Autodesk Fusion 360 part; units mm, degrees
(part 5 of 6)
sketch "Gear Tooth (2)" plane through (0, 0, 0) normal (0, 0, 1) x (1, 0, 0)
  spline S0 degree 5 poles (33.47, -4.9149) (33.4943, -4.9185) (33.543, -4.9249) (33.6161, -4.932) (33.714, -4.9371) (33.8368, -4.9373) (33.96, -4.9332) (34.0834, -4.9264) (34.2068, -4.9182) (34.3304, -4.9091) (34.454, -4.8988) (34.5776, -4.8871) (34.7013, -4.8735) (34.8251, -4.8577) (34.949, -4.8398) (35.0728, -4.8198) (35.1967, -4.7983) (35.3206, -4.7752) (35.4445, -4.751) (35.5683, -4.7256) (35.6921, -4.699) (35.8159, -4.6711) (35.9396, -4.6419) (36.0632, -4.6113) (36.1868, -4.5793) (36.3104, -4.5461) (36.4339, -4.5117) (36.5573, -4.4761) (36.6806, -4.4394) (36.8038, -4.4016) (36.927, -4.3627) (37.05, -4.3226) (37.173, -4.2815) (37.2958, -4.2393) (37.4185, -4.1961) (37.5411, -4.1517) (37.6636, -4.1064) (37.7859, -4.06) (37.9082, -4.0126) (38.0302, -3.9642) (38.1522, -3.9148) (38.274, -3.8645) (38.3956, -3.8132) (38.5172, -3.7609) (38.6385, -3.7077) (38.7597, -3.6535) (38.8807, -3.5984) (39.0016, -3.5424) (39.1223, -3.4854) (39.2428, -3.4276) (39.3631, -3.3689) (39.4833, -3.3092) (39.6032, -3.2487) (39.723, -3.1873) (39.8426, -3.125) (39.962, -3.0619) (40.0812, -2.9979) (40.2002, -2.9331) (40.319, -2.8674) (40.4376, -2.8009) (40.5559, -2.7335) (40.6741, -2.6653) (40.792, -2.5963) (40.9098, -2.5265) (41.0273, -2.4559) (41.1445, -2.3844) (41.2616, -2.3122) (41.3783, -2.2392) (41.4949, -2.1654) (41.6112, -2.0908) (41.7273, -2.0154) (41.82, -1.9545) (41.8894, -1.9084) (41.9356, -1.8776) (41.9587, -1.8621) knots 0 0 0 0 0 0 0.01428571 0.02857143 0.04285714 0.05714286 0.07142857 0.08571429 0.1 0.11428571 0.12857143 0.14285714 0.15714286 0.17142857 0.18571429 0.2 0.21428571 0.22857143 0.24285714 0.25714286 0.27142857 0.28571429 0.3 0.31428571 0.32857143 0.34285714 0.35714286 0.37142857 0.38571429 0.4 0.41428571 0.42857143 0.44285714 0.45714286 0.47142857 0.48571429 0.5 0.51428571 0.52857143 0.54285714 0.55714286 0.57142857 0.58571429 0.6 0.61428571 0.62857143 0.64285714 0.65714286 0.67142857 0.68571429 0.7 0.71428571 0.72857143 0.74285714 0.75714286 0.77142857 0.78571429 0.8 0.81428571 0.82857143 0.84285714 0.85714286 0.87142857 0.88571429 0.9 0.91428571 0.92857143 0.94285714 0.95714286 0.97142857 0.98571429 1 1 1 1 1 1
  spline S1 degree 5 poles (33.47, 4.9149) (33.4943, 4.9185) (33.543, 4.9249) (33.6161, 4.932) (33.714, 4.9371) (33.8368, 4.9373) (33.96, 4.9332) (34.0834, 4.9264) (34.2068, 4.9182) (34.3304, 4.9091) (34.454, 4.8988) (34.5776, 4.8871) (34.7013, 4.8735) (34.8251, 4.8577) (34.949, 4.8398) (35.0728, 4.8198) (35.1967, 4.7983) (35.3206, 4.7752) (35.4445, 4.751) (35.5683, 4.7256) (35.6921, 4.699) (35.8159, 4.6711) (35.9396, 4.6419) (36.0632, 4.6113) (36.1868, 4.5793) (36.3104, 4.5461) (36.4339, 4.5117) (36.5573, 4.4761) (36.6806, 4.4394) (36.8038, 4.4016) (36.927, 4.3627) (37.05, 4.3226) (37.173, 4.2815) (37.2958, 4.2393) (37.4185, 4.1961) (37.5411, 4.1517) (37.6636, 4.1064) (37.7859, 4.06) (37.9082, 4.0126) (38.0302, 3.9642) (38.1522, 3.9148) (38.274, 3.8645) (38.3956, 3.8132) (38.5172, 3.7609) (38.6385, 3.7077) (38.7597, 3.6535) (38.8807, 3.5984) (39.0016, 3.5424) (39.1223, 3.4854) (39.2428, 3.4276) (39.3631, 3.3689) (39.4833, 3.3092) (39.6032, 3.2487) (39.723, 3.1873) (39.8426, 3.125) (39.962, 3.0619) (40.0812, 2.9979) (40.2002, 2.9331) (40.319, 2.8674) (40.4376, 2.8009) (40.5559, 2.7335) (40.6741, 2.6653) (40.792, 2.5963) (40.9098, 2.5265) (41.0273, 2.4559) (41.1445, 2.3844) (41.2616, 2.3122) (41.3783, 2.2392) (41.4949, 2.1654) (41.6112, 2.0908) (41.7273, 2.0154) (41.82, 1.9545) (41.8894, 1.9084) (41.9356, 1.8776) (41.9587, 1.8621) knots 0 0 0 0 0 0 0.01428571 0.02857143 0.04285714 0.05714286 0.07142857 0.08571429 0.1 0.11428571 0.12857143 0.14285714 0.15714286 0.17142857 0.18571429 0.2 0.21428571 0.22857143 0.24285714 0.25714286 0.27142857 0.28571429 0.3 0.31428571 0.32857143 0.34285714 0.35714286 0.37142857 0.38571429 0.4 0.41428571 0.42857143 0.44285714 0.45714286 0.47142857 0.48571429 0.5 0.51428571 0.52857143 0.54285714 0.55714286 0.57142857 0.58571429 0.6 0.61428571 0.62857143 0.64285714 0.65714286 0.67142857 0.68571429 0.7 0.71428571 0.72857143 0.74285714 0.75714286 0.77142857 0.78571429 0.8 0.81428571 0.82857143 0.84285714 0.85714286 0.87142857 0.88571429 0.9 0.91428571 0.92857143 0.94285714 0.95714286 0.97142857 0.98571429 1 1 1 1 1 1
  arc A0 (41.9587, -1.8621) -> (41.9587, 1.8621) centre (0, 0) ccw
  line L0 (28.7398, -4.2203) -> (33.47, -4.9149)
  line L1 (28.7398, 4.2203) -> (33.47, 4.9149)
  line L2 (28.7398, -4.2203) -> (28.7398, 4.2203)
  point P0 (34.058, -4.9275)
  point P1 (34.6545, -4.8784)
  point P2 (35.2564, -4.787)
  point P3 (35.862, -4.66)
  point P4 (36.4705, -4.5009)
  point P5 (37.0809, -4.3121)
  point P6 (37.6927, -4.0952)
  point P7 (38.305, -3.8513)
  point P8 (38.9173, -3.5813)
  point P9 (39.5291, -3.286)
  point P10 (40.1396, -2.966)
  point P11 (40.7485, -2.6217)
  point P12 (41.355, -2.2536)
  point P13 (34.058, 4.9275)
  point P14 (34.6545, 4.8784)
  point P15 (35.2564, 4.787)
  point P16 (35.862, 4.66)
  point P17 (36.4705, 4.5009)
  point P18 (37.0809, 4.3121)
  point P19 (37.6927, 4.0952)
  point P20 (38.305, 3.8513)
  point P21 (38.9173, 3.5813)
  point P22 (39.5291, 3.286)
  point P23 (40.1396, 2.966)
  point P24 (40.7485, 2.6217)
  point P25 (41.355, 2.2536)
extrude "Extrude11" add sketch "Gear Tooth (2)" along normal blind 4 bodies 6
fillet "Fillet3" radius 2 2 edges at (28.7497, -4.2218, 2) (28.7497, 4.2218, 2) on bodies 6
pattern_circular "C-Pattern3" count 12 over 360 about axis through (0, 0, 0) along (0, 0, 1) of "Extrude11", "Fillet3"
sketch "Diametrial Pitch Circle (2)" plane through (0, 0, 0) normal (0, 0, 1) x (1, 0, 0)
  circle A0 centre (0, 0) radius 36 construction
sketch "Sketch15" plane through (0, 0, 0) normal (0, 0, 1) x (1, 0, 0)
  arc A0 (27.643, -8.9572) -> (28.4181, -6.0644) centre (0, 0) ccw
  arc A1 (30.6647, -4.503) -> (28.4181, -6.0644) centre (30.3741, -6.4818) ccw
  line L0 (30.6647, -4.503) -> (33.47, -4.9149)
  spline S0 degree 5 poles (33.47, -4.9149) (33.4943, -4.9185) (33.543, -4.9249) (33.6161, -4.932) (33.714, -4.9371) (33.8368, -4.9373) (33.96, -4.9332) (34.0834, -4.9264) (34.2068, -4.9182) (34.3304, -4.9091) (34.454, -4.8988) (34.5776, -4.8871) (34.7013, -4.8735) (34.8251, -4.8577) (34.949, -4.8398) (35.0728, -4.8198) (35.1967, -4.7983) (35.3206, -4.7752) (35.4445, -4.751) (35.5683, -4.7256) (35.6921, -4.699) (35.8159, -4.6711) (35.9396, -4.6419) (36.0632, -4.6113) (36.1868, -4.5793) (36.3104, -4.5461) (36.4339, -4.5117) (36.5573, -4.4761) (36.6806, -4.4394) (36.8038, -4.4016) (36.927, -4.3627) (37.05, -4.3226) (37.173, -4.2815) (37.2958, -4.2393) (37.4185, -4.1961) (37.5411, -4.1517) (37.6636, -4.1064) (37.7859, -4.06) (37.9082, -4.0126) (38.0302, -3.9642) (38.1522, -3.9148) (38.274, -3.8645) (38.3956, -3.8132) (38.5172, -3.7609) (38.6385, -3.7077) (38.7597, -3.6535) (38.8807, -3.5984) (39.0016, -3.5424) (39.1223, -3.4854) (39.2428, -3.4276) (39.3631, -3.3689) (39.4833, -3.3092) (39.6032, -3.2487) (39.723, -3.1873) (39.8426, -3.125) (39.962, -3.0619) (40.0812, -2.9979) (40.2002, -2.9331) (40.319, -2.8674) (40.4376, -2.8009) (40.5559, -2.7335) (40.6741, -2.6653) (40.792, -2.5963) (40.9098, -2.5265) (41.0273, -2.4559) (41.1445, -2.3844) (41.2616, -2.3122) (41.3783, -2.2392) (41.4949, -2.1654) (41.6112, -2.0908) (41.7273, -2.0154) (41.82, -1.9545) (41.8894, -1.9084) (41.9356, -1.8776) (41.9587, -1.8621) knots 0 0 0 0 0 0 0.01428571 0.02857143 0.04285714 0.05714286 0.07142857 0.08571429 0.1 0.11428571 0.12857143 0.14285714 0.15714286 0.17142857 0.18571429 0.2 0.21428571 0.22857143 0.24285714 0.25714286 0.27142857 0.28571429 0.3 0.31428571 0.32857143 0.34285714 0.35714286 0.37142857 0.38571429 0.4 0.41428571 0.42857143 0.44285714 0.45714286 0.47142857 0.48571429 0.5 0.51428571 0.52857143 0.54285714 0.55714286 0.57142857 0.58571429 0.6 0.61428571 0.62857143 0.64285714 0.65714286 0.67142857 0.68571429 0.7 0.71428571 0.72857143 0.74285714 0.75714286 0.77142857 0.78571429 0.8 0.81428571 0.82857143 0.84285714 0.85714286 0.87142857 0.88571429 0.9 0.91428571 0.92857143 0.94285714 0.95714286 0.97142857 0.98571429 1 1 1 1 1 1
  arc A2 (41.9587, -1.8621) -> (41.9587, 1.8621) centre (0, 0) ccw
  spline S1 degree 5 poles (41.9587, 1.8621) (41.9356, 1.8776) (41.8894, 1.9084) (41.82, 1.9545) (41.7273, 2.0154) (41.6112, 2.0908) (41.4949, 2.1654) (41.3783, 2.2392) (41.2616, 2.3122) (41.1445, 2.3844) (41.0273, 2.4559) (40.9098, 2.5265) (40.792, 2.5963) (40.6741, 2.6653) (40.5559, 2.7335) (40.4376, 2.8009) (40.319, 2.8674) (40.2002, 2.9331) (40.0812, 2.9979) (39.962, 3.0619) (39.8426, 3.125) (39.723, 3.1873) (39.6032, 3.2487) (39.4833, 3.3092) (39.3631, 3.3689) (39.2428, 3.4276) (39.1223, 3.4854) (39.0016, 3.5424) (38.8807, 3.5984) (38.7597, 3.6535) (38.6385, 3.7077) (38.5172, 3.7609) (38.3956, 3.8132) (38.274, 3.8645) (38.1522, 3.9148) (38.0302, 3.9642) (37.9082, 4.0126) (37.7859, 4.06) (37.6636, 4.1064) (37.5411, 4.1517) (37.4185, 4.1961) (37.2958, 4.2393) (37.173, 4.2815) (37.05, 4.3226) (36.927, 4.3627) (36.8038, 4.4016) (36.6806, 4.4394) (36.5573, 4.4761) (36.4339, 4.5117) (36.3104, 4.5461) (36.1868, 4.5793) (36.0632, 4.6113) (35.9396, 4.6419) (35.8159, 4.6711) (35.6921, 4.699) (35.5683, 4.7256) (35.4445, 4.751) (35.3206, 4.7752) (35.1967, 4.7983) (35.0728, 4.8198) (34.949, 4.8398) (34.8251, 4.8577) (34.7013, 4.8735) (34.5776, 4.8871) (34.454, 4.8988) (34.3304, 4.9091) (34.2068, 4.9182) (34.0834, 4.9264) (33.96, 4.9332) (33.8368, 4.9373) (33.714, 4.9371) (33.6161, 4.932) (33.543, 4.9249) (33.4943, 4.9185) (33.47, 4.9149) knots -1 -1 -1 -1 -1 -1 -0.98571429 -0.97142857 -0.95714286 -0.94285714 -0.92857143 -0.91428571 -0.9 -0.88571429 -0.87142857 -0.85714286 -0.84285714 -0.82857143 -0.81428571 -0.8 -0.78571429 -0.77142857 -0.75714286 -0.74285714 -0.72857143 -0.71428571 -0.7 -0.68571429 -0.67142857 -0.65714286 -0.64285714 -0.62857143 -0.61428571 -0.6 -0.58571429 -0.57142857 -0.55714286 -0.54285714 -0.52857143 -0.51428571 -0.5 -0.48571429 -0.47142857 -0.45714286 -0.44285714 -0.42857143 -0.41428571 -0.4 -0.38571429 -0.37142857 -0.35714286 -0.34285714 -0.32857143 -0.31428571 -0.3 -0.28571429 -0.27142857 -0.25714286 -0.24285714 -0.22857143 -0.21428571 -0.2 -0.18571429 -0.17142857 -0.15714286 -0.14285714 -0.12857143 -0.11428571 -0.1 -0.08571429 -0.07142857 -0.05714286 -0.04285714 -0.02857143 -0.01428571 0 0 0 0 0 0
  line L1 (33.47, 4.9149) -> (30.6647, 4.503)
  arc A3 (28.4181, 6.0644) -> (30.6647, 4.503) centre (30.3741, 6.4818) ccw
  arc A4 (28.4181, 6.0644) -> (27.643, 8.9572) centre (0, 0) ccw
  arc A5 (28.8079, 11.4326) -> (27.643, 8.9572) centre (29.5456, 9.5737) ccw
  line L2 (28.8079, 11.4326) -> (31.4433, 12.4785)
  spline S2 degree 5 poles (31.4433, 12.4785) (31.4662, 12.4876) (31.5115, 12.5064) (31.5784, 12.5368) (31.6657, 12.5814) (31.7722, 12.6426) (31.8768, 12.7077) (31.9803, 12.7753) (32.0831, 12.8441) (32.1855, 12.9138) (32.2874, 12.9845) (32.3887, 13.0565) (32.489, 13.1301) (32.5883, 13.2057) (32.6866, 13.2831) (32.7839, 13.3623) (32.8804, 13.443) (32.9762, 13.5248) (33.0713, 13.6077) (33.1659, 13.6917) (33.2598, 13.7766) (33.353, 13.8626) (33.4455, 13.9498) (33.5373, 14.0381) (33.6284, 14.1276) (33.7188, 14.2182) (33.8085, 14.3097) (33.8976, 14.4022) (33.986, 14.4957) (34.0738, 14.5901) (34.161, 14.6853) (34.2476, 14.7815) (34.3335, 14.8786) (34.4188, 14.9765) (34.5034, 15.0753) (34.5874, 15.175) (34.6708, 15.2756) (34.7536, 15.3769) (34.8357, 15.4791) (34.9173, 15.582) (34.9982, 15.6857) (35.0785, 15.7902) (35.1582, 15.8955) (35.2373, 16.0015) (35.3158, 16.1083) (35.3936, 16.2158) (35.4709, 16.324) (35.5475, 16.433) (35.6236, 16.5427) (35.699, 16.653) (35.7739, 16.764) (35.8481, 16.8758) (35.9218, 16.9882) (35.9948, 17.1012) (36.0672, 17.2149) (36.1391, 17.3293) (36.2103, 17.4443) (36.2809, 17.56) (36.351, 17.6763) (36.4204, 17.7932) (36.4892, 17.9107) (36.5575, 18.0288) (36.6251, 18.1475) (36.6921, 18.2669) (36.7586, 18.3868) (36.8244, 18.5073) (36.8897, 18.6283) (36.9543, 18.75) (37.0183, 18.8722) (37.0818, 18.995) (37.1446, 19.1183) (37.1944, 19.2174) (37.2315, 19.292) (37.2561, 19.3418) (37.2683, 19.3667) knots 0 0 0 0 0 0 0.01428571 0.02857143 0.04285714 0.05714286 0.07142857 0.08571429 0.1 0.11428571 0.12857143 0.14285714 0.15714286 0.17142857 0.18571429 0.2 0.21428571 0.22857143 0.24285714 0.25714286 0.27142857 0.28571429 0.3 0.31428571 0.32857143 0.34285714 0.35714286 0.37142857 0.38571429 0.4 0.41428571 0.42857143 0.44285714 0.45714286 0.47142857 0.48571429 0.5 0.51428571 0.52857143 0.54285714 0.55714286 0.57142857 0.58571429 0.6 0.61428571 0.62857143 0.64285714 0.65714286 0.67142857 0.68571429 0.7 0.71428571 0.72857143 0.74285714 0.75714286 0.77142857 0.78571429 0.8 0.81428571 0.82857143 0.84285714 0.85714286 0.87142857 0.88571429 0.9 0.91428571 0.92857143 0.94285714 0.95714286 0.97142857 0.98571429 1 1 1 1 1 1
  arc A6 (37.2683, 19.3667) -> (35.4063, 22.592) centre (0, 0) ccw
  spline S3 degree 5 poles (35.4063, 22.592) (35.3785, 22.5938) (35.3231, 22.5974) (35.2399, 22.6026) (35.1292, 22.609) (34.991, 22.6163) (34.853, 22.6227) (34.7151, 22.6284) (34.5774, 22.6332) (34.44, 22.6372) (34.3027, 22.6405) (34.1656, 22.6429) (34.0288, 22.6445) (33.8921, 22.6453) (33.7557, 22.6453) (33.6195, 22.6444) (33.4836, 22.6427) (33.3479, 22.6402) (33.2124, 22.6369) (33.0772, 22.6327) (32.9422, 22.6277) (32.8075, 22.6218) (32.6731, 22.6151) (32.5389, 22.6075) (32.405, 22.5991) (32.2714, 22.5898) (32.1382, 22.5796) (32.0052, 22.5686) (31.8725, 22.5567) (31.7401, 22.5439) (31.6081, 22.5302) (31.4764, 22.5156) (31.345, 22.5001) (31.214, 22.4837) (31.0833, 22.4664) (30.9531, 22.4482) (30.8231, 22.4291) (30.6936, 22.409) (30.5644, 22.388) (30.4357, 22.3661) (30.3073, 22.3432) (30.1794, 22.3193) (30.0519, 22.2944) (29.9249, 22.2685) (29.7984, 22.2417) (29.6723, 22.2138) (29.5467, 22.1849) (29.4215, 22.155) (29.2968, 22.1242) (29.1727, 22.0922) (29.0491, 22.0592) (28.926, 22.0251) (28.8036, 21.9898) (28.6819, 21.9532) (28.5608, 21.9155) (28.4403, 21.8767) (28.3203, 21.8367) (28.2009, 21.7958) (28.0821, 21.7538) (27.964, 21.7105) (27.8468, 21.6658) (27.7306, 21.6195) (27.6155, 21.5713) (27.5016, 21.5212) (27.3886, 21.4695) (27.2765, 21.4166) (27.1649, 21.3627) (27.0539, 21.3081) (26.9436, 21.2522) (26.8349, 21.1942) (26.7287, 21.1326) (26.6464, 21.0793) (26.5866, 21.0365) (26.5477, 21.0067) (26.5284, 20.9915) knots -1 -1 -1 -1 -1 -1 -0.98571429 -0.97142857 -0.95714286 -0.94285714 -0.92857143 -0.91428571 -0.9 -0.88571429 -0.87142857 -0.85714286 -0.84285714 -0.82857143 -0.81428571 -0.8 -0.78571429 -0.77142857 -0.75714286 -0.74285714 -0.72857143 -0.71428571 -0.7 -0.68571429 -0.67142857 -0.65714286 -0.64285714 -0.62857143 -0.61428571 -0.6 -0.58571429 -0.57142857 -0.55714286 -0.54285714 -0.52857143 -0.51428571 -0.5 -0.48571429 -0.47142857 -0.45714286 -0.44285714 -0.42857143 -0.41428571 -0.4 -0.38571429 -0.37142857 -0.35714286 -0.34285714 -0.32857143 -0.31428571 -0.3 -0.28571429 -0.27142857 -0.25714286 -0.24285714 -0.22857143 -0.21428571 -0.2 -0.18571429 -0.17142857 -0.15714286 -0.14285714 -0.12857143 -0.11428571 -0.1 -0.08571429 -0.07142857 -0.05714286 -0.04285714 -0.02857143 -0.01428571 0 0 0 0 0 0
  line L3 (26.5284, 20.9915) -> (24.3049, 19.232)
  arc A7 (21.5786, 19.461) -> (24.3049, 19.232) centre (23.0639, 20.8004) ccw
  arc A8 (21.5786, 19.461) -> (19.461, 21.5786) centre (0, 0) ccw
  arc A9 (19.232, 24.3049) -> (19.461, 21.5786) centre (20.8004, 23.0639) ccw
  line L4 (19.232, 24.3049) -> (20.9915, 26.5284)
  spline S4 degree 5 poles (20.9915, 26.5284) (21.0067, 26.5477) (21.0365, 26.5866) (21.0793, 26.6464) (21.1326, 26.7287) (21.1942, 26.8349) (21.2522, 26.9436) (21.3081, 27.0539) (21.3627, 27.1649) (21.4166, 27.2765) (21.4695, 27.3886) (21.5212, 27.5016) (21.5713, 27.6155) (21.6195, 27.7306) (21.6658, 27.8468) (21.7105, 27.964) (21.7538, 28.0821) (21.7958, 28.2009) (21.8367, 28.3203) (21.8767, 28.4403) (21.9155, 28.5608) (21.9532, 28.6819) (21.9898, 28.8036) (22.0251, 28.926) (22.0592, 29.0491) (22.0922, 29.1727) (22.1242, 29.2968) (22.155, 29.4215) (22.1849, 29.5467) (22.2138, 29.6723) (22.2417, 29.7984) (22.2685, 29.9249) (22.2944, 30.0519) (22.3193, 30.1794) (22.3432, 30.3073) (22.3661, 30.4357) (22.388, 30.5644) (22.409, 30.6936) (22.4291, 30.8231) (22.4482, 30.9531) (22.4664, 31.0833) (22.4837, 31.214) (22.5001, 31.345) (22.5156, 31.4764) (22.5302, 31.6081) (22.5439, 31.7401) (22.5567, 31.8725) (22.5686, 32.0052) (22.5796, 32.1382) (22.5898, 32.2714) (22.5991, 32.405) (22.6075, 32.5389) (22.6151, 32.6731) (22.6218, 32.8075) (22.6277, 32.9422) (22.6327, 33.0772) (22.6369, 33.2124) (22.6402, 33.3479) (22.6427, 33.4836) (22.6444, 33.6195) (22.6453, 33.7557) (22.6453, 33.8921) (22.6445, 34.0288) (22.6429, 34.1656) (22.6405, 34.3027) (22.6372, 34.44) (22.6332, 34.5774) (22.6284, 34.7151) (22.6227, 34.853) (22.6163, 34.991) (22.609, 35.1292) (22.6026, 35.2399) (22.5974, 35.3231) (22.5938, 35.3785) (22.592, 35.4063) knots 0 0 0 0 0 0 0.01428571 0.02857143 0.04285714 0.05714286 0.07142857 0.08571429 0.1 0.11428571 0.12857143 0.14285714 0.15714286 0.17142857 0.18571429 0.2 0.21428571 0.22857143 0.24285714 0.25714286 0.27142857 0.28571429 0.3 0.31428571 0.32857143 0.34285714 0.35714286 0.37142857 0.38571429 0.4 0.41428571 0.42857143 0.44285714 0.45714286 0.47142857 0.48571429 0.5 0.51428571 0.52857143 0.54285714 0.55714286 0.57142857 0.58571429 0.6 0.61428571 0.62857143 0.64285714 0.65714286 0.67142857 0.68571429 0.7 0.71428571 0.72857143 0.74285714 0.75714286 0.77142857 0.78571429 0.8 0.81428571 0.82857143 0.84285714 0.85714286 0.87142857 0.88571429 0.9 0.91428571 0.92857143 0.94285714 0.95714286 0.97142857 0.98571429 1 1 1 1 1 1
  arc A10 (22.592, 35.4063) -> (19.3667, 37.2683) centre (0, 0) ccw
  spline S5 degree 5 poles (19.3667, 37.2683) (19.3418, 37.2561) (19.292, 37.2315) (19.2174, 37.1944) (19.1183, 37.1446) (18.995, 37.0818) (18.8722, 37.0183) (18.75, 36.9543) (18.6283, 36.8897) (18.5073, 36.8244) (18.3868, 36.7586) (18.2669, 36.6921) (18.1475, 36.6251) (18.0288, 36.5575) (17.9107, 36.4892) (17.7932, 36.4204) (17.6763, 36.351) (17.56, 36.2809) (17.4443, 36.2103) (17.3293, 36.1391) (17.2149, 36.0672) (17.1012, 35.9948) (16.9882, 35.9218) (16.8758, 35.8481) (16.764, 35.7739) (16.653, 35.699) (16.5427, 35.6236) (16.433, 35.5475) (16.324, 35.4709) (16.2158, 35.3936) (16.1083, 35.3158) (16.0015, 35.2373) (15.8955, 35.1582) (15.7902, 35.0785) (15.6857, 34.9982) (15.582, 34.9173) (15.4791, 34.8357) (15.3769, 34.7536) (15.2756, 34.6708) (15.175, 34.5874) (15.0753, 34.5034) (14.9765, 34.4188) (14.8786, 34.3335) (14.7815, 34.2476) (14.6853, 34.161) (14.5901, 34.0738) (14.4957, 33.986) (14.4022, 33.8976) (14.3097, 33.8085) (14.2182, 33.7188) (14.1276, 33.6284) (14.0381, 33.5373) (13.9498, 33.4455) (13.8626, 33.353) (13.7766, 33.2598) (13.6917, 33.1659) (13.6077, 33.0713) (13.5248, 32.9762) (13.443, 32.8804) (13.3623, 32.7839) (13.2831, 32.6866) (13.2057, 32.5883) (13.1301, 32.489) (13.0565, 32.3887) (12.9845, 32.2874) (12.9138, 32.1855) (12.8441, 32.0831) (12.7753, 31.9803) (12.7077, 31.8768) (12.6426, 31.7722) (12.5814, 31.6657) (12.5368, 31.5784) (12.5064, 31.5115) (12.4876, 31.4662) (12.4785, 31.4433) knots -1 -1 -1 -1 -1 -1 -0.98571429 -0.97142857 -0.95714286 -0.94285714 -0.92857143 -0.91428571 -0.9 -0.88571429 -0.87142857 -0.85714286 -0.84285714 -0.82857143 -0.81428571 -0.8 -0.78571429 -0.77142857 -0.75714286 -0.74285714 -0.72857143 -0.71428571 -0.7 -0.68571429 -0.67142857 -0.65714286 -0.64285714 -0.62857143 -0.61428571 -0.6 -0.58571429 -0.57142857 -0.55714286 -0.54285714 -0.52857143 -0.51428571 -0.5 -0.48571429 -0.47142857 -0.45714286 -0.44285714 -0.42857143 -0.41428571 -0.4 -0.38571429 -0.37142857 -0.35714286 -0.34285714 -0.32857143 -0.31428571 -0.3 -0.28571429 -0.27142857 -0.25714286 -0.24285714 -0.22857143 -0.21428571 -0.2 -0.18571429 -0.17142857 -0.15714286 -0.14285714 -0.12857143 -0.11428571 -0.1 -0.08571429 -0.07142857 -0.05714286 -0.04285714 -0.02857143 -0.01428571 0 0 0 0 0 0
  line L5 (12.4785, 31.4433) -> (11.4326, 28.8079)
  arc A11 (8.9572, 27.643) -> (11.4326, 28.8079) centre (9.5737, 29.5456) ccw
  arc A12 (8.9572, 27.643) -> (6.0644, 28.4181) centre (0, 0) ccw
  arc A13 (4.503, 30.6647) -> (6.0644, 28.4181) centre (6.4818, 30.3741) ccw
  line L6 (4.503, 30.6647) -> (4.9149, 33.47)
  spline S6 degree 5 poles (4.9149, 33.47) (4.9185, 33.4943) (4.9249, 33.543) (4.932, 33.6161) (4.9371, 33.714) (4.9373, 33.8368) (4.9332, 33.96) (4.9264, 34.0834) (4.9182, 34.2068) (4.9091, 34.3304) (4.8988, 34.454) (4.8871, 34.5776) (4.8735, 34.7013) (4.8577, 34.8251) (4.8398, 34.949) (4.8198, 35.0728) (4.7983, 35.1967) (4.7752, 35.3206) (4.751, 35.4445) (4.7256, 35.5683) (4.699, 35.6921) (4.6711, 35.8159) (4.6419, 35.9396) (4.6113, 36.0632) (4.5793, 36.1868) (4.5461, 36.3104) (4.5117, 36.4339) (4.4761, 36.5573) (4.4394, 36.6806) (4.4016, 36.8038) (4.3627, 36.927) (4.3226, 37.05) (4.2815, 37.173) (4.2393, 37.2958) (4.1961, 37.4185) (4.1517, 37.5411) (4.1064, 37.6636) (4.06, 37.7859) (4.0126, 37.9082) (3.9642, 38.0302) (3.9148, 38.1522) (3.8645, 38.274) (3.8132, 38.3956) (3.7609, 38.5172) (3.7077, 38.6385) (3.6535, 38.7597) (3.5984, 38.8807) (3.5424, 39.0016) (3.4854, 39.1223) (3.4276, 39.2428) (3.3689, 39.3631) (3.3092, 39.4833) (3.2487, 39.6032) (3.1873, 39.723) (3.125, 39.8426) (3.0619, 39.962) (2.9979, 40.0812) (2.9331, 40.2002) (2.8674, 40.319) (2.8009, 40.4376) (2.7335, 40.5559) (2.6653, 40.6741) (2.5963, 40.792) (2.5265, 40.9098) (2.4559, 41.0273) (2.3844, 41.1445) (2.3122, 41.2616) (2.2392, 41.3783) (2.1654, 41.4949) (2.0908, 41.6112) (2.0154, 41.7273) (1.9545, 41.82) (1.9084, 41.8894) (1.8776, 41.9356) (1.8621, 41.9587) knots 0 0 0 0 0 0 0.01428571 0.02857143 0.04285714 0.05714286 0.07142857 0.08571429 0.1 0.11428571 0.12857143 0.14285714 0.15714286 0.17142857 0.18571429 0.2 0.21428571 0.22857143 0.24285714 0.25714286 0.27142857 0.28571429 0.3 0.31428571 0.32857143 0.34285714 0.35714286 0.37142857 0.38571429 0.4 0.41428571 0.42857143 0.44285714 0.45714286 0.47142857 0.48571429 0.5 0.51428571 0.52857143 0.54285714 0.55714286 0.57142857 0.58571429 0.6 0.61428571 0.62857143 0.64285714 0.65714286 0.67142857 0.68571429 0.7 0.71428571 0.72857143 0.74285714 0.75714286 0.77142857 0.78571429 0.8 0.81428571 0.82857143 0.84285714 0.85714286 0.87142857 0.88571429 0.9 0.91428571 0.92857143 0.94285714 0.95714286 0.97142857 0.98571429 1 1 1 1 1 1
  arc A14 (1.8621, 41.9587) -> (-1.8621, 41.9587) centre (0, 0) ccw
  spline S7 degree 5 poles (-1.8621, 41.9587) (-1.8776, 41.9356) (-1.9084, 41.8894) (-1.9545, 41.82) (-2.0154, 41.7273) (-2.0908, 41.6112) (-2.1654, 41.4949) (-2.2392, 41.3783) (-2.3122, 41.2616) (-2.3844, 41.1445) (-2.4559, 41.0273) (-2.5265, 40.9098) (-2.5963, 40.792) (-2.6653, 40.6741) (-2.7335, 40.5559) (-2.8009, 40.4376) (-2.8674, 40.319) (-2.9331, 40.2002) (-2.9979, 40.0812) (-3.0619, 39.962) (-3.125, 39.8426) (-3.1873, 39.723) (-3.2487, 39.6032) (-3.3092, 39.4833) (-3.3689, 39.3631) (-3.4276, 39.2428) (-3.4854, 39.1223) (-3.5424, 39.0016) (-3.5984, 38.8807) (-3.6535, 38.7597) (-3.7077, 38.6385) (-3.7609, 38.5172) (-3.8132, 38.3956) (-3.8645, 38.274) (-3.9148, 38.1522) (-3.9642, 38.0302) (-4.0126, 37.9082) (-4.06, 37.7859) (-4.1064, 37.6636) (-4.1517, 37.5411) (-4.1961, 37.4185) (-4.2393, 37.2958) (-4.2815, 37.173) (-4.3226, 37.05) (-4.3627, 36.927) (-4.4016, 36.8038) (-4.4394, 36.6806) (-4.4761, 36.5573) (-4.5117, 36.4339) (-4.5461, 36.3104) (-4.5793, 36.1868) (-4.6113, 36.0632) (-4.6419, 35.9396) (-4.6711, 35.8159) (-4.699, 35.6921) (-4.7256, 35.5683) (-4.751, 35.4445) (-4.7752, 35.3206) (-4.7983, 35.1967) (-4.8198, 35.0728) (-4.8398, 34.949) (-4.8577, 34.8251) (-4.8735, 34.7013) (-4.8871, 34.5776) (-4.8988, 34.454) (-4.9091, 34.3304) (-4.9182, 34.2068) (-4.9264, 34.0834) (-4.9332, 33.96) (-4.9373, 33.8368) (-4.9371, 33.714) (-4.932, 33.6161) (-4.9249, 33.543) (-4.9185, 33.4943) (-4.9149, 33.47) knots -1 -1 -1 -1 -1 -1 -0.98571429 -0.97142857 -0.95714286 -0.94285714 -0.92857143 -0.91428571 -0.9 -0.88571429 -0.87142857 -0.85714286 -0.84285714 -0.82857143 -0.81428571 -0.8 -0.78571429 -0.77142857 -0.75714286 -0.74285714 -0.72857143 -0.71428571 -0.7 -0.68571429 -0.67142857 -0.65714286 -0.64285714 -0.62857143 -0.61428571 -0.6 -0.58571429 -0.57142857 -0.55714286 -0.54285714 -0.52857143 -0.51428571 -0.5 -0.48571429 -0.47142857 -0.45714286 -0.44285714 -0.42857143 -0.41428571 -0.4 -0.38571429 -0.37142857 -0.35714286 -0.34285714 -0.32857143 -0.31428571 -0.3 -0.28571429 -0.27142857 -0.25714286 -0.24285714 -0.22857143 -0.21428571 -0.2 -0.18571429 -0.17142857 -0.15714286 -0.14285714 -0.12857143 -0.11428571 -0.1 -0.08571429 -0.07142857 -0.05714286 -0.04285714 -0.02857143 -0.01428571 0 0 0 0 0 0
  line L7 (-4.9149, 33.47) -> (-4.503, 30.6647)
  arc A15 (-6.0644, 28.4181) -> (-4.503, 30.6647) centre (-6.4818, 30.3741) ccw
  arc A16 (-6.0644, 28.4181) -> (-8.9572, 27.643) centre (0, 0) ccw
  arc A17 (-11.4326, 28.8079) -> (-8.9572, 27.643) centre (-9.5737, 29.5456) ccw
  line L8 (-11.4326, 28.8079) -> (-12.4785, 31.4433)
  spline S8 degree 5 poles (-12.4785, 31.4433) (-12.4876, 31.4662) (-12.5064, 31.5115) (-12.5368, 31.5784) (-12.5814, 31.6657) (-12.6426, 31.7722) (-12.7077, 31.8768) (-12.7753, 31.9803) (-12.8441, 32.0831) (-12.9138, 32.1855) (-12.9845, 32.2874) (-13.0565, 32.3887) (-13.1301, 32.489) (-13.2057, 32.5883) (-13.2831, 32.6866) (-13.3623, 32.7839) (-13.443, 32.8804) (-13.5248, 32.9762) (-13.6077, 33.0713) (-13.6917, 33.1659) (-13.7766, 33.2598) (-13.8626, 33.353) (-13.9498, 33.4455) (-14.0381, 33.5373) (-14.1276, 33.6284) (-14.2182, 33.7188) (-14.3097, 33.8085) (-14.4022, 33.8976) (-14.4957, 33.986) (-14.5901, 34.0738) (-14.6853, 34.161) (-14.7815, 34.2476) (-14.8786, 34.3335) (-14.9765, 34.4188) (-15.0753, 34.5034) (-15.175, 34.5874) (-15.2756, 34.6708) (-15.3769, 34.7536) (-15.4791, 34.8357) (-15.582, 34.9173) (-15.6857, 34.9982) (-15.7902, 35.0785) (-15.8955, 35.1582) (-16.0015, 35.2373) (-16.1083, 35.3158) (-16.2158, 35.3936) (-16.324, 35.4709) (-16.433, 35.5475) (-16.5427, 35.6236) (-16.653, 35.699) (-16.764, 35.7739) (-16.8758, 35.8481) (-16.9882, 35.9218) (-17.1012, 35.9948) (-17.2149, 36.0672) (-17.3293, 36.1391) (-17.4443, 36.2103) (-17.56, 36.2809) (-17.6763, 36.351) (-17.7932, 36.4204) (-17.9107, 36.4892) (-18.0288, 36.5575) (-18.1475, 36.6251) (-18.2669, 36.6921) (-18.3868, 36.7586) (-18.5073, 36.8244) (-18.6283, 36.8897) (-18.75, 36.9543) (-18.8722, 37.0183) (-18.995, 37.0818) (-19.1183, 37.1446) (-19.2174, 37.1944) (-19.292, 37.2315) (-19.3418, 37.2561) (-19.3667, 37.2683) knots 0 0 0 0 0 0 0.01428571 0.02857143 0.04285714 0.05714286 0.07142857 0.08571429 0.1 0.11428571 0.12857143 0.14285714 0.15714286 0.17142857 0.18571429 0.2 0.21428571 0.22857143 0.24285714 0.25714286 0.27142857 0.28571429 0.3 0.31428571 0.32857143 0.34285714 0.35714286 0.37142857 0.38571429 0.4 0.41428571 0.42857143 0.44285714 0.45714286 0.47142857 0.48571429 0.5 0.51428571 0.52857143 0.54285714 0.55714286 0.57142857 0.58571429 0.6 0.61428571 0.62857143 0.64285714 0.65714286 0.67142857 0.68571429 0.7 0.71428571 0.72857143 0.74285714 0.75714286 0.77142857 0.78571429 0.8 0.81428571 0.82857143 0.84285714 0.85714286 0.87142857 0.88571429 0.9 0.91428571 0.92857143 0.94285714 0.95714286 0.97142857 0.98571429 1 1 1 1 1 1
  arc A18 (-19.3667, 37.2683) -> (-22.592, 35.4063) centre (0, 0) ccw
  spline S9 degree 5 poles (-22.592, 35.4063) (-22.5938, 35.3785) (-22.5974, 35.3231) (-22.6026, 35.2399) (-22.609, 35.1292) (-22.6163, 34.991) (-22.6227, 34.853) (-22.6284, 34.7151) (-22.6332, 34.5774) (-22.6372, 34.44) (-22.6405, 34.3027) (-22.6429, 34.1656) (-22.6445, 34.0288) (-22.6453, 33.8921) (-22.6453, 33.7557) (-22.6444, 33.6195) (-22.6427, 33.4836) (-22.6402, 33.3479) (-22.6369, 33.2124) (-22.6327, 33.0772) (-22.6277, 32.9422) (-22.6218, 32.8075) (-22.6151, 32.6731) (-22.6075, 32.5389) (-22.5991, 32.405) (-22.5898, 32.2714) (-22.5796, 32.1382) (-22.5686, 32.0052) (-22.5567, 31.8725) (-22.5439, 31.7401) (-22.5302, 31.6081) (-22.5156, 31.4764) (-22.5001, 31.345) (-22.4837, 31.214) (-22.4664, 31.0833) (-22.4482, 30.9531) (-22.4291, 30.8231) (-22.409, 30.6936) (-22.388, 30.5644) (-22.3661, 30.4357) (-22.3432, 30.3073) (-22.3193, 30.1794) (-22.2944, 30.0519) (-22.2685, 29.9249) (-22.2417, 29.7984) (-22.2138, 29.6723) (-22.1849, 29.5467) (-22.155, 29.4215) (-22.1242, 29.2968) (-22.0922, 29.1727) (-22.0592, 29.0491) (-22.0251, 28.926) (-21.9898, 28.8036) (-21.9532, 28.6819) (-21.9155, 28.5608) (-21.8767, 28.4403) (-21.8367, 28.3203) (-21.7958, 28.2009) (-21.7538, 28.0821) (-21.7105, 27.964) (-21.6658, 27.8468) (-21.6195, 27.7306) (-21.5713, 27.6155) (-21.5212, 27.5016) (-21.4695, 27.3886) (-21.4166, 27.2765) (-21.3627, 27.1649) (-21.3081, 27.0539) (-21.2522, 26.9436) (-21.1942, 26.8349) (-21.1326, 26.7287) (-21.0793, 26.6464) (-21.0365, 26.5866) (-21.0067, 26.5477) (-20.9915, 26.5284) knots -1 -1 -1 -1 -1 -1 -0.98571429 -0.97142857 -0.95714286 -0.94285714 -0.92857143 -0.91428571 -0.9 -0.88571429 -0.87142857 -0.85714286 -0.84285714 -0.82857143 -0.81428571 -0.8 -0.78571429 -0.77142857 -0.75714286 -0.74285714 -0.72857143 -0.71428571 -0.7 -0.68571429 -0.67142857 -0.65714286 -0.64285714 -0.62857143 -0.61428571 -0.6 -0.58571429 -0.57142857 -0.55714286 -0.54285714 -0.52857143 -0.51428571 -0.5 -0.48571429 -0.47142857 -0.45714286 -0.44285714 -0.42857143 -0.41428571 -0.4 -0.38571429 -0.37142857 -0.35714286 -0.34285714 -0.32857143 -0.31428571 -0.3 -0.28571429 -0.27142857 -0.25714286 -0.24285714 -0.22857143 -0.21428571 -0.2 -0.18571429 -0.17142857 -0.15714286 -0.14285714 -0.12857143 -0.11428571 -0.1 -0.08571429 -0.07142857 -0.05714286 -0.04285714 -0.02857143 -0.01428571 0 0 0 0 0 0
  line L9 (-20.9915, 26.5284) -> (-19.232, 24.3049)
  arc A19 (-19.461, 21.5786) -> (-19.232, 24.3049) centre (-20.8004, 23.0639) ccw
  arc A20 (-19.461, 21.5786) -> (-21.5786, 19.461) centre (0, 0) ccw
  arc A21 (-24.3049, 19.232) -> (-21.5786, 19.461) centre (-23.0639, 20.8004) ccw
  line L10 (-24.3049, 19.232) -> (-26.5284, 20.9915)
  spline S10 degree 5 poles (-26.5284, 20.9915) (-26.5477, 21.0067) (-26.5866, 21.0365) (-26.6464, 21.0793) (-26.7287, 21.1326) (-26.8349, 21.1942) (-26.9436, 21.2522) (-27.0539, 21.3081) (-27.1649, 21.3627) (-27.2765, 21.4166) (-27.3886, 21.4695) (-27.5016, 21.5212) (-27.6155, 21.5713) (-27.7306, 21.6195) (-27.8468, 21.6658) (-27.964, 21.7105) (-28.0821, 21.7538) (-28.2009, 21.7958) (-28.3203, 21.8367) (-28.4403, 21.8767) (-28.5608, 21.9155) (-28.6819, 21.9532) (-28.8036, 21.9898) (-28.926, 22.0251) (-29.0491, 22.0592) (-29.1727, 22.0922) (-29.2968, 22.1242) (-29.4215, 22.155) (-29.5467, 22.1849) (-29.6723, 22.2138) (-29.7984, 22.2417) (-29.9249, 22.2685) (-30.0519, 22.2944) (-30.1794, 22.3193) (-30.3073, 22.3432) (-30.4357, 22.3661) (-30.5644, 22.388) (-30.6936, 22.409) (-30.8231, 22.4291) (-30.9531, 22.4482) (-31.0833, 22.4664) (-31.214, 22.4837) (-31.345, 22.5001) (-31.4764, 22.5156) (-31.6081, 22.5302) (-31.7401, 22.5439) (-31.8725, 22.5567) (-32.0052, 22.5686) (-32.1382, 22.5796) (-32.2714, 22.5898) (-32.405, 22.5991) (-32.5389, 22.6075) (-32.6731, 22.6151) (-32.8075, 22.6218) (-32.9422, 22.6277) (-33.0772, 22.6327) (-33.2124, 22.6369) (-33.3479, 22.6402) (-33.4836, 22.6427) (-33.6195, 22.6444) (-33.7557, 22.6453) (-33.8921, 22.6453) (-34.0288, 22.6445) (-34.1656, 22.6429) (-34.3027, 22.6405) (-34.44, 22.6372) (-34.5774, 22.6332) (-34.7151, 22.6284) (-34.853, 22.6227) (-34.991, 22.6163) (-35.1292, 22.609) (-35.2399, 22.6026) (-35.3231, 22.5974) (-35.3785, 22.5938) (-35.4063, 22.592) knots 0 0 0 0 0 0 0.01428571 0.02857143 0.04285714 0.05714286 0.07142857 0.08571429 0.1 0.11428571 0.12857143 0.14285714 0.15714286 0.17142857 0.18571429 0.2 0.21428571 0.22857143 0.24285714 0.25714286 0.27142857 0.28571429 0.3 0.31428571 0.32857143 0.34285714 0.35714286 0.37142857 0.38571429 0.4 0.41428571 0.42857143 0.44285714 0.45714286 0.47142857 0.48571429 0.5 0.51428571 0.52857143 0.54285714 0.55714286 0.57142857 0.58571429 0.6 0.61428571 0.62857143 0.64285714 0.65714286 0.67142857 0.68571429 0.7 0.71428571 0.72857143 0.74285714 0.75714286 0.77142857 0.78571429 0.8 0.81428571 0.82857143 0.84285714 0.85714286 0.87142857 0.88571429 0.9 0.91428571 0.92857143 0.94285714 0.95714286 0.97142857 0.98571429 1 1 1 1 1 1
  arc A22 (-35.4063, 22.592) -> (-37.2683, 19.3667) centre (0, 0) ccw
  spline S11 degree 5 poles (-37.2683, 19.3667) (-37.2561, 19.3418) (-37.2315, 19.292) (-37.1944, 19.2174) (-37.1446, 19.1183) (-37.0818, 18.995) (-37.0183, 18.8722) (-36.9543, 18.75) (-36.8897, 18.6283) (-36.8244, 18.5073) (-36.7586, 18.3868) (-36.6921, 18.2669) (-36.6251, 18.1475) (-36.5575, 18.0288) (-36.4892, 17.9107) (-36.4204, 17.7932) (-36.351, 17.6763) (-36.2809, 17.56) (-36.2103, 17.4443) (-36.1391, 17.3293) (-36.0672, 17.2149) (-35.9948, 17.1012) (-35.9218, 16.9882) (-35.8481, 16.8758) (-35.7739, 16.764) (-35.699, 16.653) (-35.6236, 16.5427) (-35.5475, 16.433) (-35.4709, 16.324) (-35.3936, 16.2158) (-35.3158, 16.1083) (-35.2373, 16.0015) (-35.1582, 15.8955) (-35.0785, 15.7902) (-34.9982, 15.6857) (-34.9173, 15.582) (-34.8357, 15.4791) (-34.7536, 15.3769) (-34.6708, 15.2756) (-34.5874, 15.175) (-34.5034, 15.0753) (-34.4188, 14.9765) (-34.3335, 14.8786) (-34.2476, 14.7815) (-34.161, 14.6853) (-34.0738, 14.5901) (-33.986, 14.4957) (-33.8976, 14.4022) (-33.8085, 14.3097) (-33.7188, 14.2182) (-33.6284, 14.1276) (-33.5373, 14.0381) (-33.4455, 13.9498) (-33.353, 13.8626) (-33.2598, 13.7766) (-33.1659, 13.6917) (-33.0713, 13.6077) (-32.9762, 13.5248) (-32.8804, 13.443) (-32.7839, 13.3623) (-32.6866, 13.2831) (-32.5883, 13.2057) (-32.489, 13.1301) (-32.3887, 13.0565) (-32.2874, 12.9845) (-32.1855, 12.9138) (-32.0831, 12.8441) (-31.9803, 12.7753) (-31.8768, 12.7077) (-31.7722, 12.6426) (-31.6657, 12.5814) (-31.5784, 12.5368) (-31.5115, 12.5064) (-31.4662, 12.4876) (-31.4433, 12.4785) knots -1 -1 -1 -1 -1 -1 -0.98571429 -0.97142857 -0.95714286 -0.94285714 -0.92857143 -0.91428571 -0.9 -0.88571429 -0.87142857 -0.85714286 -0.84285714 -0.82857143 -0.81428571 -0.8 -0.78571429 -0.77142857 -0.75714286 -0.74285714 -0.72857143 -0.71428571 -0.7 -0.68571429 -0.67142857 -0.65714286 -0.64285714 -0.62857143 -0.61428571 -0.6 -0.58571429 -0.57142857 -0.55714286 -0.54285714 -0.52857143 -0.51428571 -0.5 -0.48571429 -0.47142857 -0.45714286 -0.44285714 -0.42857143 -0.41428571 -0.4 -0.38571429 -0.37142857 -0.35714286 -0.34285714 -0.32857143 -0.31428571 -0.3 -0.28571429 -0.27142857 -0.25714286 -0.24285714 -0.22857143 -0.21428571 -0.2 -0.18571429 -0.17142857 -0.15714286 -0.14285714 -0.12857143 -0.11428571 -0.1 -0.08571429 -0.07142857 -0.05714286 -0.04285714 -0.02857143 -0.01428571 0 0 0 0 0 0
  line L11 (-31.4433, 12.4785) -> (-28.8079, 11.4326)
  arc A23 (-27.643, 8.9572) -> (-28.8079, 11.4326) centre (-29.5456, 9.5737) ccw
  arc A24 (-27.643, 8.9572) -> (-28.4181, 6.0644) centre (0, 0) ccw
  arc A25 (-30.6647, 4.503) -> (-28.4181, 6.0644) centre (-30.3741, 6.4818) ccw
  line L12 (-30.6647, 4.503) -> (-33.47, 4.9149)
  spline S12 degree 5 poles (-33.47, 4.9149) (-33.4943, 4.9185) (-33.543, 4.9249) (-33.6161, 4.932) (-33.714, 4.9371) (-33.8368, 4.9373) (-33.96, 4.9332) (-34.0834, 4.9264) (-34.2068, 4.9182) (-34.3304, 4.9091) (-34.454, 4.8988) (-34.5776, 4.8871) (-34.7013, 4.8735) (-34.8251, 4.8577) (-34.949, 4.8398) (-35.0728, 4.8198) (-35.1967, 4.7983) (-35.3206, 4.7752) (-35.4445, 4.751) (-35.5683, 4.7256) (-35.6921, 4.699) (-35.8159, 4.6711) (-35.9396, 4.6419) (-36.0632, 4.6113) (-36.1868, 4.5793) (-36.3104, 4.5461) (-36.4339, 4.5117) (-36.5573, 4.4761) (-36.6806, 4.4394) (-36.8038, 4.4016) (-36.927, 4.3627) (-37.05, 4.3226) (-37.173, 4.2815) (-37.2958, 4.2393) (-37.4185, 4.1961) (-37.5411, 4.1517) (-37.6636, 4.1064) (-37.7859, 4.06) (-37.9082, 4.0126) (-38.0302, 3.9642) (-38.1522, 3.9148) (-38.274, 3.8645) (-38.3956, 3.8132) (-38.5172, 3.7609) (-38.6385, 3.7077) (-38.7597, 3.6535) (-38.8807, 3.5984) (-39.0016, 3.5424) (-39.1223, 3.4854) (-39.2428, 3.4276) (-39.3631, 3.3689) (-39.4833, 3.3092) (-39.6032, 3.2487) (-39.723, 3.1873) (-39.8426, 3.125) (-39.962, 3.0619) (-40.0812, 2.9979) (-40.2002, 2.9331) (-40.319, 2.8674) (-40.4376, 2.8009) (-40.5559, 2.7335) (-40.6741, 2.6653) (-40.792, 2.5963) (-40.9098, 2.5265) (-41.0273, 2.4559) (-41.1445, 2.3844) (-41.2616, 2.3122) (-41.3783, 2.2392) (-41.4949, 2.1654) (-41.6112, 2.0908) (-41.7273, 2.0154) (-41.82, 1.9545) (-41.8894, 1.9084) (-41.9356, 1.8776) (-41.9587, 1.8621) knots 0 0 0 0 0 0 0.01428571 0.02857143 0.04285714 0.05714286 0.07142857 0.08571429 0.1 0.11428571 0.12857143 0.14285714 0.15714286 0.17142857 0.18571429 0.2 0.21428571 0.22857143 0.24285714 0.25714286 0.27142857 0.28571429 0.3 0.31428571 0.32857143 0.34285714 0.35714286 0.37142857 0.38571429 0.4 0.41428571 0.42857143 0.44285714 0.45714286 0.47142857 0.48571429 0.5 0.51428571 0.52857143 0.54285714 0.55714286 0.57142857 0.58571429 0.6 0.61428571 0.62857143 0.64285714 0.65714286 0.67142857 0.68571429 0.7 0.71428571 0.72857143 0.74285714 0.75714286 0.77142857 0.78571429 0.8 0.81428571 0.82857143 0.84285714 0.85714286 0.87142857 0.88571429 0.9 0.91428571 0.92857143 0.94285714 0.95714286 0.97142857 0.98571429 1 1 1 1 1 1
  arc A26 (-41.9587, 1.8621) -> (-41.9587, -1.8621) centre (0, 0) ccw
  spline S13 degree 5 poles (-41.9587, -1.8621) (-41.9356, -1.8776) (-41.8894, -1.9084) (-41.82, -1.9545) (-41.7273, -2.0154) (-41.6112, -2.0908) (-41.4949, -2.1654) (-41.3783, -2.2392) (-41.2616, -2.3122) (-41.1445, -2.3844) (-41.0273, -2.4559) (-40.9098, -2.5265) (-40.792, -2.5963) (-40.6741, -2.6653) (-40.5559, -2.7335) (-40.4376, -2.8009) (-40.319, -2.8674) (-40.2002, -2.9331) (-40.0812, -2.9979) (-39.962, -3.0619) (-39.8426, -3.125) (-39.723, -3.1873) (-39.6032, -3.2487) (-39.4833, -3.3092) (-39.3631, -3.3689) (-39.2428, -3.4276) (-39.1223, -3.4854) (-39.0016, -3.5424) (-38.8807, -3.5984) (-38.7597, -3.6535) (-38.6385, -3.7077) (-38.5172, -3.7609) (-38.3956, -3.8132) (-38.274, -3.8645) (-38.1522, -3.9148) (-38.0302, -3.9642) (-37.9082, -4.0126) (-37.7859, -4.06) (-37.6636, -4.1064) (-37.5411, -4.1517) (-37.4185, -4.1961) (-37.2958, -4.2393) (-37.173, -4.2815) (-37.05, -4.3226) (-36.927, -4.3627) (-36.8038, -4.4016) (-36.6806, -4.4394) (-36.5573, -4.4761) (-36.4339, -4.5117) (-36.3104, -4.5461) (-36.1868, -4.5793) (-36.0632, -4.6113) (-35.9396, -4.6419) (-35.8159, -4.6711) (-35.6921, -4.699) (-35.5683, -4.7256) (-35.4445, -4.751) (-35.3206, -4.7752) (-35.1967, -4.7983) (-35.0728, -4.8198) (-34.949, -4.8398) (-34.8251, -4.8577) (-34.7013, -4.8735) (-34.5776, -4.8871) (-34.454, -4.8988) (-34.3304, -4.9091) (-34.2068, -4.9182) (-34.0834, -4.9264) (-33.96, -4.9332) (-33.8368, -4.9373) (-33.714, -4.9371) (-33.6161, -4.932) (-33.543, -4.9249) (-33.4943, -4.9185) (-33.47, -4.9149) knots -1 -1 -1 -1 -1 -1 -0.98571429 -0.97142857 -0.95714286 -0.94285714 -0.92857143 -0.91428571 -0.9 -0.88571429 -0.87142857 -0.85714286 -0.84285714 -0.82857143 -0.81428571 -0.8 -0.78571429 -0.77142857 -0.75714286 -0.74285714 -0.72857143 -0.71428571 -0.7 -0.68571429 -0.67142857 -0.65714286 -0.64285714 -0.62857143 -0.61428571 -0.6 -0.58571429 -0.57142857 -0.55714286 -0.54285714 -0.52857143 -0.51428571 -0.5 -0.48571429 -0.47142857 -0.45714286 -0.44285714 -0.42857143 -0.41428571 -0.4 -0.38571429 -0.37142857 -0.35714286 -0.34285714 -0.32857143 -0.31428571 -0.3 -0.28571429 -0.27142857 -0.25714286 -0.24285714 -0.22857143 -0.21428571 -0.2 -0.18571429 -0.17142857 -0.15714286 -0.14285714 -0.12857143 -0.11428571 -0.1 -0.08571429 -0.07142857 -0.05714286 -0.04285714 -0.02857143 -0.01428571 0 0 0 0 0 0
  line L13 (-33.47, -4.9149) -> (-30.6647, -4.503)
  arc A27 (-28.4181, -6.0644) -> (-30.6647, -4.503) centre (-30.3741, -6.4818) ccw
  arc A28 (-28.4181, -6.0644) -> (-27.643, -8.9572) centre (0, 0) ccw
  arc A29 (-28.8079, -11.4326) -> (-27.643, -8.9572) centre (-29.5456, -9.5737) ccw
  line L14 (-28.8079, -11.4326) -> (-31.4433, -12.4785)
  spline S14 degree 5 poles (-31.4433, -12.4785) (-31.4662, -12.4876) (-31.5115, -12.5064) (-31.5784, -12.5368) (-31.6657, -12.5814) (-31.7722, -12.6426) (-31.8768, -12.7077) (-31.9803, -12.7753) (-32.0831, -12.8441) (-32.1855, -12.9138) (-32.2874, -12.9845) (-32.3887, -13.0565) (-32.489, -13.1301) (-32.5883, -13.2057) (-32.6866, -13.2831) (-32.7839, -13.3623) (-32.8804, -13.443) (-32.9762, -13.5248) (-33.0713, -13.6077) (-33.1659, -13.6917) (-33.2598, -13.7766) (-33.353, -13.8626) (-33.4455, -13.9498) (-33.5373, -14.0381) (-33.6284, -14.1276) (-33.7188, -14.2182) (-33.8085, -14.3097) (-33.8976, -14.4022) (-33.986, -14.4957) (-34.0738, -14.5901) (-34.161, -14.6853) (-34.2476, -14.7815) (-34.3335, -14.8786) (-34.4188, -14.9765) (-34.5034, -15.0753) (-34.5874, -15.175) (-34.6708, -15.2756) (-34.7536, -15.3769) (-34.8357, -15.4791) (-34.9173, -15.582) (-34.9982, -15.6857) (-35.0785, -15.7902) (-35.1582, -15.8955) (-35.2373, -16.0015) (-35.3158, -16.1083) (-35.3936, -16.2158) (-35.4709, -16.324) (-35.5475, -16.433) (-35.6236, -16.5427) (-35.699, -16.653) (-35.7739, -16.764) (-35.8481, -16.8758) (-35.9218, -16.9882) (-35.9948, -17.1012) (-36.0672, -17.2149) (-36.1391, -17.3293) (-36.2103, -17.4443) (-36.2809, -17.56) (-36.351, -17.6763) (-36.4204, -17.7932) (-36.4892, -17.9107) (-36.5575, -18.0288) (-36.6251, -18.1475) (-36.6921, -18.2669) (-36.7586, -18.3868) (-36.8244, -18.5073) (-36.8897, -18.6283) (-36.9543, -18.75) (-37.0183, -18.8722) (-37.0818, -18.995) (-37.1446, -19.1183) (-37.1944, -19.2174) (-37.2315, -19.292) (-37.2561, -19.3418) (-37.2683, -19.3667) knots 0 0 0 0 0 0 0.01428571 0.02857143 0.04285714 0.05714286 0.07142857 0.08571429 0.1 0.11428571 0.12857143 0.14285714 0.15714286 0.17142857 0.18571429 0.2 0.21428571 0.22857143 0.24285714 0.25714286 0.27142857 0.28571429 0.3 0.31428571 0.32857143 0.34285714 0.35714286 0.37142857 0.38571429 0.4 0.41428571 0.42857143 0.44285714 0.45714286 0.47142857 0.48571429 0.5 0.51428571 0.52857143 0.54285714 0.55714286 0.57142857 0.58571429 0.6 0.61428571 0.62857143 0.64285714 0.65714286 0.67142857 0.68571429 0.7 0.71428571 0.72857143 0.74285714 0.75714286 0.77142857 0.78571429 0.8 0.81428571 0.82857143 0.84285714 0.85714286 0.87142857 0.88571429 0.9 0.91428571 0.92857143 0.94285714 0.95714286 0.97142857 0.98571429 1 1 1 1 1 1
  arc A30 (-37.2683, -19.3667) -> (-35.4063, -22.592) centre (0, 0) ccw
  spline S15 degree 5 poles (-35.4063, -22.592) (-35.3785, -22.5938) (-35.3231, -22.5974) (-35.2399, -22.6026) (-35.1292, -22.609) (-34.991, -22.6163) (-34.853, -22.6227) (-34.7151, -22.6284) (-34.5774, -22.6332) (-34.44, -22.6372) (-34.3027, -22.6405) (-34.1656, -22.6429) (-34.0288, -22.6445) (-33.8921, -22.6453) (-33.7557, -22.6453) (-33.6195, -22.6444) (-33.4836, -22.6427) (-33.3479, -22.6402) (-33.2124, -22.6369) (-33.0772, -22.6327) (-32.9422, -22.6277) (-32.8075, -22.6218) (-32.6731, -22.6151) (-32.5389, -22.6075) (-32.405, -22.5991) (-32.2714, -22.5898) (-32.1382, -22.5796) (-32.0052, -22.5686) (-31.8725, -22.5567) (-31.7401, -22.5439) (-31.6081, -22.5302) (-31.4764, -22.5156) (-31.345, -22.5001) (-31.214, -22.4837) (-31.0833, -22.4664) (-30.9531, -22.4482) (-30.8231, -22.4291) (-30.6936, -22.409) (-30.5644, -22.388) (-30.4357, -22.3661) (-30.3073, -22.3432) (-30.1794, -22.3193) (-30.0519, -22.2944) (-29.9249, -22.2685) (-29.7984, -22.2417) (-29.6723, -22.2138) (-29.5467, -22.1849) (-29.4215, -22.155) (-29.2968, -22.1242) (-29.1727, -22.0922) (-29.0491, -22.0592) (-28.926, -22.0251) (-28.8036, -21.9898) (-28.6819, -21.9532) (-28.5608, -21.9155) (-28.4403, -21.8767) (-28.3203, -21.8367) (-28.2009, -21.7958) (-28.0821, -21.7538) (-27.964, -21.7105) (-27.8468, -21.6658) (-27.7306, -21.6195) (-27.6155, -21.5713) (-27.5016, -21.5212) (-27.3886, -21.4695) (-27.2765, -21.4166) (-27.1649, -21.3627) (-27.0539, -21.3081) (-26.9436, -21.2522) (-26.8349, -21.1942) (-26.7287, -21.1326) (-26.6464, -21.0793) (-26.5866, -21.0365) (-26.5477, -21.0067) (-26.5284, -20.9915) knots -1 -1 -1 -1 -1 -1 -0.98571429 -0.97142857 -0.95714286 -0.94285714 -0.92857143 -0.91428571 -0.9 -0.88571429 -0.87142857 -0.85714286 -0.84285714 -0.82857143 -0.81428571 -0.8 -0.78571429 -0.77142857 -0.75714286 -0.74285714 -0.72857143 -0.71428571 -0.7 -0.68571429 -0.67142857 -0.65714286 -0.64285714 -0.62857143 -0.61428571 -0.6 -0.58571429 -0.57142857 -0.55714286 -0.54285714 -0.52857143 -0.51428571 -0.5 -0.48571429 -0.47142857 -0.45714286 -0.44285714 -0.42857143 -0.41428571 -0.4 -0.38571429 -0.37142857 -0.35714286 -0.34285714 -0.32857143 -0.31428571 -0.3 -0.28571429 -0.27142857 -0.25714286 -0.24285714 -0.22857143 -0.21428571 -0.2 -0.18571429 -0.17142857 -0.15714286 -0.14285714 -0.12857143 -0.11428571 -0.1 -0.08571429 -0.07142857 -0.05714286 -0.04285714 -0.02857143 -0.01428571 0 0 0 0 0 0
  line L15 (-26.5284, -20.9915) -> (-24.3049, -19.232)
  arc A31 (-21.5786, -19.461) -> (-24.3049, -19.232) centre (-23.0639, -20.8004) ccw
  arc A32 (-21.5786, -19.461) -> (-19.461, -21.5786) centre (0, 0) ccw
  arc A33 (-19.232, -24.3049) -> (-19.461, -21.5786) centre (-20.8004, -23.0639) ccw
  line L16 (-19.232, -24.3049) -> (-20.9915, -26.5284)
  spline S16 degree 5 poles (-20.9915, -26.5284) (-21.0067, -26.5477) (-21.0365, -26.5866) (-21.0793, -26.6464) (-21.1326, -26.7287) (-21.1942, -26.8349) (-21.2522, -26.9436) (-21.3081, -27.0539) (-21.3627, -27.1649) (-21.4166, -27.2765) (-21.4695, -27.3886) (-21.5212, -27.5016) (-21.5713, -27.6155) (-21.6195, -27.7306) (-21.6658, -27.8468) (-21.7105, -27.964) (-21.7538, -28.0821) (-21.7958, -28.2009) (-21.8367, -28.3203) (-21.8767, -28.4403) (-21.9155, -28.5608) (-21.9532, -28.6819) (-21.9898, -28.8036) (-22.0251, -28.926) (-22.0592, -29.0491) (-22.0922, -29.1727) (-22.1242, -29.2968) (-22.155, -29.4215) (-22.1849, -29.5467) (-22.2138, -29.6723) (-22.2417, -29.7984) (-22.2685, -29.9249) (-22.2944, -30.0519) (-22.3193, -30.1794) (-22.3432, -30.3073) (-22.3661, -30.4357) (-22.388, -30.5644) (-22.409, -30.6936) (-22.4291, -30.8231) (-22.4482, -30.9531) (-22.4664, -31.0833) (-22.4837, -31.214) (-22.5001, -31.345) (-22.5156, -31.4764) (-22.5302, -31.6081) (-22.5439, -31.7401) (-22.5567, -31.8725) (-22.5686, -32.0052) (-22.5796, -32.1382) (-22.5898, -32.2714) (-22.5991, -32.405) (-22.6075, -32.5389) (-22.6151, -32.6731) (-22.6218, -32.8075) (-22.6277, -32.9422) (-22.6327, -33.0772) (-22.6369, -33.2124) (-22.6402, -33.3479) (-22.6427, -33.4836) (-22.6444, -33.6195) (-22.6453, -33.7557) (-22.6453, -33.8921) (-22.6445, -34.0288) (-22.6429, -34.1656) (-22.6405, -34.3027) (-22.6372, -34.44) (-22.6332, -34.5774) (-22.6284, -34.7151) (-22.6227, -34.853) (-22.6163, -34.991) (-22.609, -35.1292) (-22.6026, -35.2399) (-22.5974, -35.3231) (-22.5938, -35.3785) (-22.592, -35.4063) knots 0 0 0 0 0 0 0.01428571 0.02857143 0.04285714 0.05714286 0.07142857 0.08571429 0.1 0.11428571 0.12857143 0.14285714 0.15714286 0.17142857 0.18571429 0.2 0.21428571 0.22857143 0.24285714 0.25714286 0.27142857 0.28571429 0.3 0.31428571 0.32857143 0.34285714 0.35714286 0.37142857 0.38571429 0.4 0.41428571 0.42857143 0.44285714 0.45714286 0.47142857 0.48571429 0.5 0.51428571 0.52857143 0.54285714 0.55714286 0.57142857 0.58571429 0.6 0.61428571 0.62857143 0.64285714 0.65714286 0.67142857 0.68571429 0.7 0.71428571 0.72857143 0.74285714 0.75714286 0.77142857 0.78571429 0.8 0.81428571 0.82857143 0.84285714 0.85714286 0.87142857 0.88571429 0.9 0.91428571 0.92857143 0.94285714 0.95714286 0.97142857 0.98571429 1 1 1 1 1 1
  arc A34 (-22.592, -35.4063) -> (-19.3667, -37.2683) centre (0, 0) ccw
  spline S17 degree 5 poles (-19.3667, -37.2683) (-19.3418, -37.2561) (-19.292, -37.2315) (-19.2174, -37.1944) (-19.1183, -37.1446) (-18.995, -37.0818) (-18.8722, -37.0183) (-18.75, -36.9543) (-18.6283, -36.8897) (-18.5073, -36.8244) (-18.3868, -36.7586) (-18.2669, -36.6921) (-18.1475, -36.6251) (-18.0288, -36.5575) (-17.9107, -36.4892) (-17.7932, -36.4204) (-17.6763, -36.351) (-17.56, -36.2809) (-17.4443, -36.2103) (-17.3293, -36.1391) (-17.2149, -36.0672) (-17.1012, -35.9948) (-16.9882, -35.9218) (-16.8758, -35.8481) (-16.764, -35.7739) (-16.653, -35.699) (-16.5427, -35.6236) (-16.433, -35.5475) (-16.324, -35.4709) (-16.2158, -35.3936) (-16.1083, -35.3158) (-16.0015, -35.2373) (-15.8955, -35.1582) (-15.7902, -35.0785) (-15.6857, -34.9982) (-15.582, -34.9173) (-15.4791, -34.8357) (-15.3769, -34.7536) (-15.2756, -34.6708) (-15.175, -34.5874) (-15.0753, -34.5034) (-14.9765, -34.4188) (-14.8786, -34.3335) (-14.7815, -34.2476) (-14.6853, -34.161) (-14.5901, -34.0738) (-14.4957, -33.986) (-14.4022, -33.8976) (-14.3097, -33.8085) (-14.2182, -33.7188) (-14.1276, -33.6284) (-14.0381, -33.5373) (-13.9498, -33.4455) (-13.8626, -33.353) (-13.7766, -33.2598) (-13.6917, -33.1659) (-13.6077, -33.0713) (-13.5248, -32.9762) (-13.443, -32.8804) (-13.3623, -32.7839) (-13.2831, -32.6866) (-13.2057, -32.5883) (-13.1301, -32.489) (-13.0565, -32.3887) (-12.9845, -32.2874) (-12.9138, -32.1855) (-12.8441, -32.0831) (-12.7753, -31.9803) (-12.7077, -31.8768) (-12.6426, -31.7722) (-12.5814, -31.6657) (-12.5368, -31.5784) (-12.5064, -31.5115) (-12.4876, -31.4662) (-12.4785, -31.4433) knots -1 -1 -1 -1 -1 -1 -0.98571429 -0.97142857 -0.95714286 -0.94285714 -0.92857143 -0.91428571 -0.9 -0.88571429 -0.87142857 -0.85714286 -0.84285714 -0.82857143 -0.81428571 -0.8 -0.78571429 -0.77142857 -0.75714286 -0.74285714 -0.72857143 -0.71428571 -0.7 -0.68571429 -0.67142857 -0.65714286 -0.64285714 -0.62857143 -0.61428571 -0.6 -0.58571429 -0.57142857 -0.55714286 -0.54285714 -0.52857143 -0.51428571 -0.5 -0.48571429 -0.47142857 -0.45714286 -0.44285714 -0.42857143 -0.41428571 -0.4 -0.38571429 -0.37142857 -0.35714286 -0.34285714 -0.32857143 -0.31428571 -0.3 -0.28571429 -0.27142857 -0.25714286 -0.24285714 -0.22857143 -0.21428571 -0.2 -0.18571429 -0.17142857 -0.15714286 -0.14285714 -0.12857143 -0.11428571 -0.1 -0.08571429 -0.07142857 -0.05714286 -0.04285714 -0.02857143 -0.01428571 0 0 0 0 0 0
  line L17 (-12.4785, -31.4433) -> (-11.4326, -28.8079)
  arc A35 (-8.9572, -27.643) -> (-11.4326, -28.8079) centre (-9.5737, -29.5456) ccw
  arc A36 (-8.9572, -27.643) -> (-6.0644, -28.4181) centre (0, 0) ccw
  arc A37 (-4.503, -30.6647) -> (-6.0644, -28.4181) centre (-6.4818, -30.3741) ccw